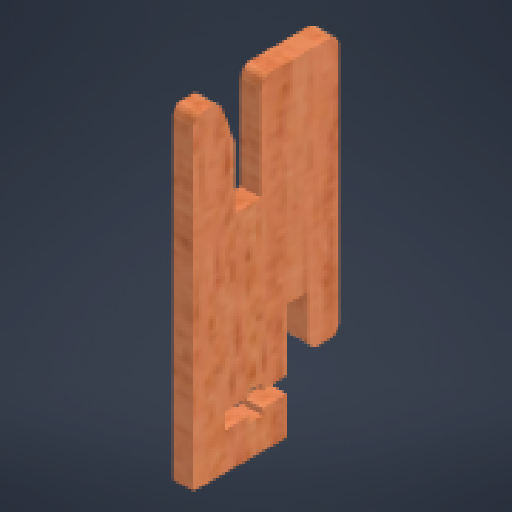
# Autodesk Inventor part: CoverHolder
Saved by Autodesk Inventor 2024.1 (Build 281209000, 209)
## iProperties
Created: 2023-05-18
Part Number: CoverHolder
Material: MDF Medium Density Fiberboard
Document SubType Name: Modeling
Designer: jaege
Density: 0.8 g/cm^3
Appearance: Red Oak - Natural Low Gloss
Author: jaege
Autodesk Inventor part; units mm, degrees
ref_plane "YZ Plane" through (0, 0, 0) normal (1, 0, 0) x (0, 1, 0)
ref_plane "XZ Plane" through (0, 0, 0) normal (0, 1, 0) x (-1, 0, 0)
ref_plane "XY Plane" through (0, 0, 0) normal (0, 0, 1) x (1, 0, 0)
sketch "Sketch1" plane through (0, 0, 0) normal (1, 0, 0) x (0, 1, 0)
  line L0 (5.1523, -6.7614) -> (5.1523, -11.7614)
  line L1 (24.8477, -15.2386) -> (24.8477, -19.2386)
  line L2 (24.8477, -19.2386) -> (-24.8477, -19.2386)
  line L3 (-24.8477, -19.2386) -> (-24.8477, -2.7614)
  line L4 (-24.8477, -2.7614) -> (-14.8477, -2.7614)
  line L5 (-14.8477, -2.7614) -> (-14.8477, 1.2386)
  line L6 (-14.8477, 1.2386) -> (-24.8477, 1.2386)
  line L7 (-24.8477, 1.2386) -> (-24.8477, 19.2386) construction
  line L8 (-24.8477, 19.2386) -> (24.8477, 19.2386)
  line L9 (24.8477, 19.2386) -> (24.8477, -6.7614)
  line L10 (24.8477, 19.2386) -> (-24.8477, -19.2386) construction
  line L11 (-24.8477, 19.2386) -> (-37.0477, 19.2386)
  line L12 (-37.0477, 19.2386) -> (-37.0477, 1.2386)
  line L13 (-37.0477, 1.2386) -> (-29.8477, 1.2386)
  line L14 (-24.8477, 1.2386) -> (-24.8477, 19.2386) construction
  line L15 (-31.0477, 8.4386) -> (-29.8477, 8.4386)
  line L16 (-25.6477, 8.4386) -> (-25.6477, 6.0386)
  line L17 (-25.6477, 6.0386) -> (-26.8477, 6.0386)
  line L18 (-31.0477, 6.0386) -> (-31.0477, 8.4386)
  line L19 (-29.8477, 13.2386) -> (-26.8477, 13.2386)
  line L20 (-26.8477, 13.2386) -> (-26.8477, 8.4386)
  line L21 (-26.8477, 1.2386) -> (-29.8477, 1.2386) construction
  line L22 (-29.8477, 1.2386) -> (-29.8477, 6.0386)
  line L23 (-29.8477, 8.4386) -> (-26.8477, 8.4386) construction
  line L24 (-29.8477, 8.4386) -> (-29.8477, 13.2386)
  line L25 (-29.8477, 6.0386) -> (-29.8477, 8.4386) construction
  line L26 (-26.8477, 8.4386) -> (-25.6477, 8.4386)
  line L27 (-26.8477, 8.4386) -> (-26.8477, 6.0386) construction
  line L28 (-26.8477, 6.0386) -> (-26.8477, 1.2386)
  line L29 (-26.8477, 6.0386) -> (-29.8477, 6.0386) construction
  line L30 (-29.8477, 6.0386) -> (-31.0477, 6.0386)
  line L31 (-29.8477, 1.2386) -> (-26.8477, 1.2386) construction
  line L32 (-26.8477, 1.2386) -> (-24.8477, 1.2386)
  line L33 (5.1523, -6.7614) -> (24.8477, -6.7614)
  line L34 (5.1523, -11.7614) -> (18.8252, -11.7614)
  line L35 (18.8252, -11.7614) -> (24.8477, -15.2386)
  point P0 (0, 0)
  point P1 (0, 0)
  point P2 (-28.3477, 13.2386)
  point P3 (-28.3477, -1.2973)
  point P4 (-31.0477, 7.2386)
  point P5 (-29.9884, 7.2386)
  dimension "d1" = 4
  dimension "d7" = 10
  dimension "d8" = 20
  dimension "d9" = 20
  dimension "d15" = 5.4
  dimension "d16" = 2.4
  dimension "d17" = 3
  dimension "d18" = 12
  dimension "d19" = 6
  dimension "d20" = 2
  dimension "d21" = 6
  dimension "d23" = 5
  dimension "d24" = 30
  dimension "d25" = 19.6954
  dimension "d26" = 4
  dimension "d27" = 4
  constraints: 72 end point, 25 parallel, 14 perpendicular, 6 horizontal, 4 point on line, 3 horizontal alignment, 3 midpoint, 2 collinear, 1 coincident, 1 vertical, 1 vertical alignment
  measures "d1" distance between parallel lines of L4 L6
  measures "d7" distance of L3.end L4.end
  measures "d8" distance between parallel lines of L0 L5
  measures "d9" distance of L0.end L1.start
  measures "d15" distance of L16.end L18.start
  measures "d16" distance of L16.start L16.end
  measures "d17" distance of L21.start L13.end
  measures "d18" distance of L19.end L21.start
  measures "d19" distance between parallel lines of L18 L12
  measures "d20" distance between parallel lines of L3 L20
  measures "d21" distance between parallel lines of L11 L19
  measures "d23" distance of L0.start L0.end
  measures "d24" angle of L34 L35
  measures "d25" distance of L0.start L9.end
  measures "d26" distance of L1.start L1.end
  measures "d27" distance between parallel lines of L4 L33
extrude "Extrusion1" add sketch "Sketch1" along normal blind 4
fillet "Fillet1" radius 2 9 edges at (2, 24.8477, 19.2386) (2, 24.8477, -6.7614) (2, -24.8477, -2.7614) (2, -24.8477, -19.2386) (2, 24.8477, -15.2386) (2, 24.8477, -19.2386) (2, -37.0477, 19.2386) (2, 18.8252, -11.7614) (2, -37.0477, 1.2386)
body "Solid1"
